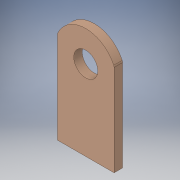
# Autodesk Inventor part: mdf_support
Saved by Autodesk Inventor 2018 (Build 220112000, 112)
## iProperties
Created: 2018-09-09
Part Number: mdf_support
Material: Generic
Document SubType Name: Modeling
Designer: Fredy Espana C
Density: 1 g/cm^3
Appearance: Default
Author: Fredy Espana C
Autodesk Inventor part; units mm, degrees
ref_plane "YZ Plane" through (0, 0, 0) normal (1, 0, 0) x (0, 1, 0)
ref_plane "XZ Plane" through (0, 0, 0) normal (0, 1, 0) x (-1, 0, 0)
ref_plane "XY Plane" through (0, 0, 0) normal (0, 0, 1) x (1, 0, 0)
sketch "Sketch1" plane through (0, 0, 0) normal (0, 0, 1) x (1, 0, 0)
  circle A0 centre (0, 0) radius 8.5
  line L0 (20, 8.5) -> (20, -56.5)
  line L1 (20, -56.5) -> (-20, -56.5)
  line L2 (-20, -56.5) -> (-20, 8.5)
  arc A1 (20, 8.5) -> (-20, 8.5) centre (0, 0) ccw
  point P0 (0, 8.5)
  dimension "d0" = 17
  dimension "d1" = 65
  dimension "d3" = 20
  dimension "d4" = 8.5
  constraints: 6 end point, 2 coincident, 2 parallel, 2 point on circle, 1 centre point, 1 horizontal alignment, 1 perpendicular, 1 vertical, 1 vertical alignment, 2 other
  measures "d1" distance of L0.start L0.end
  measures "d3" distance from line of point (0, 0) L2
  measures "d4" distance of point (0, 0) point (0, 8.5)
extrude "Extrusion1" add sketch "Sketch1" along normal blind 6
fillet "Fillet1" radius 3 2 edges at (20, 8.5, 3) (-20, 8.5, 3)
body "Solid1"
